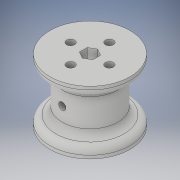
# Autodesk Inventor part: Pulley
Saved by Autodesk Inventor 2019 (Build 230136000, 136)
## iProperties
Created: 2019-02-03
Part Number: Pulley
Material: Generic
Document SubType Name: Modeling
Designer: Ashley
Density: 1 g/cm^3
Appearance: Default
Author: Ashley
Autodesk Inventor part; units mm, degrees
ref_plane "YZ Plane" through (0, 0, 0) normal (1, 0, 0) x (0, 1, 0)
ref_plane "XZ Plane" through (0, 0, 0) normal (0, 1, 0) x (-1, 0, 0)
ref_plane "XY Plane" through (0, 0, 0) normal (0, 0, 1) x (1, 0, 0)
sketch "Middle Sketch" plane through (0, 0, 0) normal (0, 1, 0) x (-1, 0, 0)
  circle A0 centre (0, 0) radius 11.5
  dimension "d0" = 23
  constraints: 1 centre point, 1 coincident
  measures "d0" diameter of A0
extrude "Middle Extrusion" add sketch "Middle Sketch" along normal mid plane 17.3333
sketch "Side Sketch" plane through (0, 8.6667, 0) normal (0, 1, 0) x (1, 0, 0)
  circle A0 centre (0, 0) radius 11.5 construction
  circle A1 centre (0, 0) radius 16.5
  dimension "d3" = 33
  constraints: 1 centre point, 1 coincident
  measures "d3" diameter of A1
extrude "Side Extrusion" add sketch "Side Sketch" along normal blind 4.3333
mirror "Side Mirror" about plane through (0, 0, 0) normal (0, 1, 0) of "Side Extrusion"
fillet "Center Smoothing" radius 3 2 edges at (-16.5, 8.6667, 0) (-16.5, -8.6667, 0)
fillet "Center Smoothing" radius 3 2 edges at (11.5, -8.6667, 0) (11.5, 8.6667, 0)
sketch "Sketch3" plane through (0, -13, 0) normal (0, -1, 0) x (1, 0, 0)
  circle A0 centre (0, 0) radius 16.5 construction
  line L0 (-2.7713, -1.6) -> (-2.7713, 1.6)
  line L1 (-2.7713, 1.6) -> (0, 3.2)
  line L2 (0, 3.2) -> (2.7713, 1.6)
  line L3 (2.7713, 1.6) -> (2.7713, -1.6)
  line L4 (2.7713, -1.6) -> (0, -3.2)
  line L5 (-2.7713, 0) -> (0, 0) construction
  line L6 (0, 0) -> (2.7713, 0) construction
  line L7 (0, 3.2) -> (0, 0) construction
  line L8 (0, 0) -> (0, -3.2) construction
  line L9 (0, -3.2) -> (-2.7713, -1.6)
  dimension "d8" = 3.2
  dimension "d10" = 3.2
  dimension "d11" = 3.2
  dimension "d12" = 3.2
  dimension "d13" = 3.2
  dimension "d15" = 120
  dimension "d16" = 120
  dimension "d17" = 120
  dimension "d18" = 120
  constraints: 20 end point, 2 midpoint, 1 collinear, 1 horizontal, 1 vertical
  measures "d8" distance of L0.start L0.end
  measures "d10" distance of L0.end L1.end
  measures "d11" distance of L1.end L2.end
  measures "d12" distance of L2.end L3.end
  measures "d13" distance of L3.end L4.end
  measures "d15" angle of L1 L0
  measures "d16" angle of L2 L1
  measures "d17" angle of L3 L2
  measures "d18" angle of L3 L4
extrude "Extrusion3" cut sketch "Sketch3" against normal up to next
sketch "Sketch4" plane through (0, -13, 0) normal (0, -1, 0) x (1, 0, 0)
  circle A0 centre (0, 0) radius 16.5 construction
  circle A1 centre (-8, 0) radius 1.675
  line L0 (0, 0) -> (-16.5, 0) construction
  circle A2 centre (0, 0) radius 16.5 construction
  circle A3 centre (0, -8) radius 1.675
  circle A4 centre (8, 0) radius 1.675
  circle A5 centre (0, 8) radius 1.675
  dimension "d22" = 3.35
  dimension "d23" = 8
  dimension "d26" = 360
  constraints: 4 centre point, 2 end point, 1 horizontal, 1 horizontal alignment, 1 point on line, 10 other
  measures "d22" diameter of A1
  measures "d23" distance of A1.centre L0.start
extrude "Extrusion4" cut sketch "Sketch4" against normal up to next
sketch "Sketch5" plane through (0, -13, 0) normal (0, -1, 0) x (1, 0, 0)
  circle A0 centre (0, 0) radius 16.5 construction
  circle A1 centre (0, 0) radius 5
  dimension "d30" = 10
  constraints: 1 centre point, 1 coincident
  measures "d30" diameter of A1
extrude "Extrusion5" cut sketch "Sketch5" against normal blind 2.9
sketch "Sketch6" plane through (0, 0, 0) normal (0, 0, 1) x (1, 0, 0)
  circle A0 centre (0, 0) radius 1.5
  dimension "d33" = 3
  constraints: 1 centre point, 1 coincident
  measures "d33" diameter of A0
extrude "Extrusion6" cut sketch "Sketch6" along normal through all both and the other way through all
equation "\"d0\" = MidD"
equation "\"d1\" = MidL"
equation "\"d3\" = OuterD"
equation "\"d4\" = OuterL"
equation "\"d20\" = OuterD"
equation "\"d28\" = OuterD"
equation "\"MidD\" = 23"
equation "\"OuterD\" = 33"
equation "\"Length\" = 26"
equation "\"MidL\" = Length - 2 * OuterL"
equation "\"OuterL\" = 0.166667 * Length"
body "Solid1"
